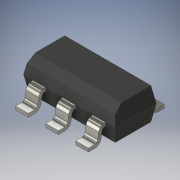
# Autodesk Inventor part: Semiconductor_SOT23-6
Saved by Autodesk Inventor 2018 (Build 220112000, 112)
## iProperties
Created: 2016-08-15
Part Number: Semiconductor_SOT23-6
Material: ABS Plastic
Document SubType Name: Modeling
Designer: Bradley
Density: 1.06 g/cm^3
Appearance: Smooth - Black
Author: Bradley
Autodesk Inventor part; units mm, degrees
ref_plane "YZ Plane" through (0, 0, 0) normal (1, 0, 0) x (0, 1, 0)
ref_plane "XZ Plane" through (0, 0, 0) normal (0, 1, 0) x (-1, 0, 0)
ref_plane "XY Plane" through (0, 0, 0) normal (0, 0, 1) x (1, 0, 0)
sketch "Sketch1" plane through (0, 0, 0) normal (0, 1, 0) x (-1, 0, 0)
  line L0 (-1.45, 0.65) -> (1.45, 0.65)
  line L1 (1.45, 0.65) -> (1.45, -0.65)
  line L2 (1.45, -0.65) -> (-1.45, -0.65)
  line L3 (-1.45, -0.65) -> (-1.45, 0.65)
  line L4 (-1.45, 0.65) -> (1.45, -0.65) construction
  line L5 (1.45, 0.65) -> (-1.45, -0.65) construction
  point P0 (0, 0)
  dimension "d0" = 2.9
  dimension "d1" = 1.3
  constraints: 12 end point, 2 midpoint, 2 parallel, 1 horizontal, 1 perpendicular
  measures "d0" distance of L1.end L2.end
  measures "d1" distance of L0.end L1.end
extrude "Extrusion1" add sketch "Sketch1" along normal blind 0.5 draft -10
sketch "Sketch2" plane through (0, 0, 0) normal (0, -1, 0) x (1, 0, 0)
  line L0 (1.45, 0.65) -> (-1.45, 0.65) projected
  line L1 (-1.45, 0.65) -> (-1.45, -0.65) projected
  line L2 (-1.45, -0.65) -> (1.45, -0.65) projected
  line L3 (1.45, -0.65) -> (1.45, 0.65) projected
  point P0 (0, 0)
extrude "Extrusion2" add sketch "Sketch2" along normal blind 0.5 draft -10
sketch "Sketch3" plane through (0, 0, 0) normal (0, 1, 0) x (-1, 0, 0)
  line L0 (-1.45, 0.65) -> (1.45, 0.65) projected
  line L1 (1.45, 0.65) -> (1.45, -0.65) projected
  line L2 (1.45, -0.65) -> (-1.45, -0.65) projected
  line L3 (-1.45, -0.65) -> (-1.45, 0.65) projected
  line L4 (-1.15, 0.65) -> (-0.75, 0.65)
  line L5 (-0.75, 0.65) -> (-0.75, 0.67)
  line L6 (-0.75, 0.67) -> (-1.15, 0.67)
  line L7 (-1.15, 0.67) -> (-1.15, 0.65)
  line L8 (-0.2, -0.65) -> (0.2, -0.65)
  line L9 (0.2, -0.65) -> (0.2, -0.67)
  line L10 (0.2, -0.67) -> (-0.2, -0.67)
  line L11 (-0.2, -0.67) -> (-0.2, -0.65)
  line L12 (-0.75, 0.65) -> (-1.15, 0.65)
  line L13 (-1.15, 0.65) -> (-1.15, 0)
  line L14 (-1.15, 0) -> (-0.75, 0)
  line L15 (-0.75, 0) -> (-0.75, 0.65)
  line L16 (-0.2, -0.65) -> (0.2, -0.65)
  line L17 (0.2, -0.65) -> (0.2, 0)
  line L18 (0.2, 0) -> (-0.2, 0)
  line L19 (-0.2, 0) -> (-0.2, -0.65)
  point P0 (0, 0)
  point P1 (0, -0.67)
  point P2 (-0.95, 0.67)
  point P3 (0, 0)
  dimension "d6" = 0.4
  dimension "d7" = 0.02
  dimension "d8" = 0.95
  dimension "d9" = 0
  constraints: 32 end point, 10 parallel, 4 horizontal, 4 perpendicular, 3 midpoint, 2 horizontal alignment, 2 point on line
  measures "d6" distance of L5.end L6.end
  measures "d7" distance of L4.end L5.end
  measures "d8" horizontal distance of point (-0.95, 0.67) point (0, 0)
  measures "d9" horizontal distance of point (0, 0) point (0, -0.67)
extrude "Extrusion3" add sketch "Sketch3" against normal blind 0.11 contours L7 L6 L5 L0 | L0 L15 L14 L13
sketch "Sketch4" plane through (1.15, 0, 0.67) normal (1, 0, 0) x (0, 0, -1)
  line L0 (0.02, 0) -> (0.0394, -0.11) projected
  line L1 (0, 0) -> (0.02, 0) projected
  line L2 (0, 0) -> (0, -0.11) projected
  line L3 (0.0394, -0.11) -> (0, -0.11) projected
  line L4 (0, -0.11) -> (0.0394, -0.11) projected
  arc A0 (0, -0.11) -> (-0.0985, -0.193) centre (0, -0.21) ccw
  arc A1 (0, 0) -> (-0.207, -0.1744) centre (0, -0.21) ccw
  arc A2 (-0.337, -0.44) -> (-0.2384, -0.357) centre (-0.337, -0.34) ccw
  arc A3 (-0.337, -0.55) -> (-0.13, -0.3756) centre (-0.337, -0.34) ccw
  line L5 (-0.0985, -0.193) -> (-0.13, -0.3756)
  line L6 (-0.207, -0.1744) -> (-0.2384, -0.357)
  line L7 (-0.337, -0.44) -> (-0.53, -0.44)
  line L8 (-0.53, -0.44) -> (-0.53, -0.55)
  line L9 (-0.53, -0.55) -> (-0.337, -0.55)
  line L10 (0.0394, -0.11) -> (0, -0.11) projected
  line L11 (0, 0) -> (0.02, 0) projected
  line L12 (0, 0) -> (0, -0.11) projected
  line L13 (1.2318, -0.5) -> (0.1082, -0.5) projected
  point P0 (0.67, 0)
  dimension "d12" = 1.2
  dimension "d13" = 0.05
  dimension "d14" = 0.1
  dimension "d15" = 0.4
  constraints: 10 end point, 8 point on circle, 8 tangent, 4 centre point, 2 coincident, 2 parallel, 2 perpendicular, 1 equal radius, 1 horizontal
  measures "d12" distance from line of point (0.67, 0) L8
  measures "d13" distance between parallel lines of L9 L13
  measures "d14" radius of A0
  measures "d15" distance from line of L5.end L8
extrude "Extrusion4" add sketch "Sketch4" against normal up to surface (0.4 mm away) contours L2 A0 L5 A3 L9 L8 L7 A2 L6 A1
extrude "Extrusion5" add sketch "Sketch3" against normal blind 0.11 contours L19 L18 L17 L2 | L2 L9 L10 L11
sketch "Sketch5" plane through (0.2, 0, -0.65) normal (1, 0, 0) x (0, 0, -1)
  line L0 (-1.3, 0) -> (-1.2806, -0.11) projected
  line L1 (-1.32, 0) -> (-1.3, 0) projected
  arc A0 (-1.32, 0) -> (-1.527, -0.1744) centre (-1.32, -0.21) ccw projected
  line L2 (-1.527, -0.1744) -> (-1.5584, -0.357) projected
  arc A1 (-1.657, -0.44) -> (-1.5584, -0.357) centre (-1.657, -0.34) ccw projected
  line L3 (-1.657, -0.44) -> (-1.85, -0.44) projected
  line L4 (-1.85, -0.44) -> (-1.85, -0.55) projected
  line L5 (-1.85, -0.55) -> (-1.657, -0.55) projected
  arc A2 (-1.657, -0.55) -> (-1.45, -0.3756) centre (-1.657, -0.34) ccw projected
  line L6 (-1.45, -0.3756) -> (-1.4185, -0.193) projected
  arc A3 (-1.32, -0.11) -> (-1.4185, -0.193) centre (-1.32, -0.21) ccw projected
  line L7 (-1.2806, -0.11) -> (-1.32, -0.11) projected
  line L8 (-0.0194, -0.11) -> (0, 0) projected
  line L9 (0.02, -0.11) -> (-0.0194, -0.11) projected
  line L10 (0.02, 0) -> (0.02, -0.11) projected
  line L11 (0, 0) -> (0.02, 0) projected
  arc A4 (0.1185, -0.193) -> (0.02, -0.11) centre (0.02, -0.21) ccw
  line L12 (0.02, 0) -> (0, 0) projected
  arc A5 (0.227, -0.1744) -> (0.02, 0) centre (0.02, -0.21) ccw
  arc A6 (0.2584, -0.357) -> (0.357, -0.44) centre (0.357, -0.34) ccw
  arc A7 (0.15, -0.3756) -> (0.357, -0.55) centre (0.357, -0.34) ccw
  line L13 (0.357, -0.55) -> (0.55, -0.55)
  line L14 (0.55, -0.55) -> (0.55, -0.44)
  line L15 (0.55, -0.44) -> (0.357, -0.44)
  line L16 (0.227, -0.1744) -> (0.2584, -0.357)
  line L17 (0.1185, -0.193) -> (0.15, -0.3756)
  point P0 (-0.65, 0)
  constraints: 10 end point, 8 point on circle, 7 tangent, 5 equal length, 4 centre point, 4 equal radius, 2 perpendicular, 1 collinear, 1 horizontal
extrude "Extrusion6" add sketch "Sketch5" against normal up to surface (0.4 mm away) contours L10 A5 L16 A6 L15 L14 L13 A7 L17 A4
pattern_linear "Rectangular Pattern1" count 3 spacing 0.95 along (-1, 0, 0) of "Extrusion3", "Extrusion4"
pattern_linear "Rectangular Pattern2" count 3 spacing 0.95 along (1, 0, 0) of "Extrusion6", "Extrusion5" first direction both ways yes
chamfer "Chamfer1" distance 0.2 angle 45 1 edges at (0, 0.5, 0.5618)
body "Solid1"
